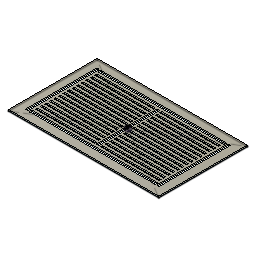
top half mount v2 (Autodesk Fusion 360 design; units mm, degrees)
Autodesk Fusion 360 part; units mm, degrees
sketch "Sketch1" plane through (0, 0, 0) normal (0, 0, 1) x (1, 0, 0)
  line L0 (115.5, -68.05) -> (-115.5, -68.05)
  line L1 (-115.5, -68.05) -> (-115.5, 68.05)
  line L2 (-115.5, 68.05) -> (115.5, 68.05)
  line L3 (115.5, 68.05) -> (115.5, -68.05)
  line L4 (115.5, -68.05) -> (-115.5, 68.05) construction
  line L5 (-115.5, -68.05) -> (115.5, 68.05) construction
  dimension "d1" = 136.1
  dimension "d2" = 231
  constraint horizontal L0
  constraint perpendicular L0 L1
  constraint parallel L0 L2
  constraint parallel L1 L3
  constraint coincident L4 origin
  constraint coincident L5 origin
  measures "d1" distance of L0.end L1.end
  measures "d2" distance of L0.start L0.end
extrude "Extrude1" add sketch "Sketch1" along normal blind 2
sketch "Sketch2" plane through (0, 0, 2) normal (0, 0, 1) x (-1, 0, 0)
  line L0 (-115.5, -68.05) -> (115.5, -68.05)
  line L1 (115.5, -68.05) -> (115.5, 68.05)
  line L2 (115.5, 68.05) -> (-115.5, 68.05)
  line L3 (-115.5, 68.05) -> (-115.5, -68.05)
  line L4 (5, -8.94) -> (95, -8.94)
  line L5 (5, -1.94) -> (95, -1.94)
  line L6 (-5, -8.94) -> (-5, -11.94)
  line L7 (2, 47) -> (-2, 47)
  line L8 (-5, -29.94) -> (-5, -32.94)
  line L9 (-5, 5.06) -> (-5, 2.06)
  line L10 (-5, -36.94) -> (-5, -39.94)
  line L11 (5, 47.06) -> (95, 47.06)
  line L12 (-5, 40.06) -> (-5, 37.06)
  line L13 (-5, 19.06) -> (-5, 16.06)
  line L14 (-95, 44.06) -> (-95, 47.06)
  arc A0 (-96, 55.06) -> (-97, 54.06) centre (-96, 54.06) ccw
  line L15 (-95, -25.94) -> (-95, -22.94)
  line L16 (-95, -39.94) -> (-95, -36.94)
  arc A1 (-100, -54.94) -> (-99, -53.94) centre (-100, -53.94) ccw
  line L17 (5, 30.06) -> (5, 33.06)
  line L18 (2, -47) -> (2, 47)
  line L19 (-95, 30.06) -> (-95, 33.06)
  line L20 (5, 44.06) -> (5, 47.06)
  arc A2 (-103, -53.94) -> (-102, -54.94) centre (-102, -53.94) ccw
  line L21 (-102, 54.94) -> (-100, 54.94)
  line L22 (5, 37.06) -> (5, 40.06)
  line L23 (-95, -46.94) -> (-95, -43.94)
  line L24 (-95.0527, 9.06) -> (-95.0527, 12.06)
  line L25 (-5, -1.94) -> (-5, -4.94)
  line L26 (5, 16.06) -> (5, 19.06)
  arc A3 (-97, -53.94) -> (-96, -54.94) centre (-96, -53.94) ccw
  line L27 (-100, -54.94) -> (-102, -54.94)
  line L28 (-95.0527, 2.06) -> (-95.0527, 5.06)
  line L29 (-97, 54.06) -> (-97, 52.06)
  line L30 (-5, -43.94) -> (-5, -46.94)
  line L31 (-97, -53.94) -> (-97, -51.94)
  line L32 (5, -4.94) -> (5, -1.94)
  line L33 (5, 23.06) -> (5, 26.06)
  line L34 (-5, -22.94) -> (-5, -25.94)
  line L35 (-2, 47) -> (-2, -47)
  line L36 (-94.8877, -18.94) -> (-94.8877, -15.94)
  line L37 (-2, 47) -> (2, -47) construction
  arc A4 (-96, -50.94) -> (-97, -51.94) centre (-96, -51.94) ccw
  line L38 (-103, -53.94) -> (-103, 53.94)
  line L39 (5, -46.94) -> (5, -43.94)
  line L40 (-95.0527, -11.94) -> (-95.0527, -8.94)
  line L41 (5, 9.06) -> (5, 12.06)
  line L42 (-95.0527, 16.06) -> (-95.0527, 19.06)
  line L43 (-95, -32.94) -> (-95, -29.94)
  line L44 (5, -39.94) -> (5, -36.94)
  line L45 (5, -18.94) -> (5, -15.94)
  arc A5 (-97, 52.06) -> (-96, 51.06) centre (-96, 52.06) ccw
  line L46 (-95, 37.06) -> (-95, 40.06)
  line L47 (-95.0527, -4.94) -> (-95.0527, -1.94)
  arc A6 (-102, 54.94) -> (-103, 53.94) centre (-102, 53.94) ccw
  line L48 (-99, 53.94) -> (-99, -53.94)
  line L49 (95, -29.94) -> (95, -32.94)
  line L50 (-94.8877, -15.94) -> (-5, -15.94)
  line L51 (-5, -25.94) -> (-95, -25.94)
  line L52 (-5, -4.94) -> (-95.0527, -4.94)
  line L53 (95, 26.06) -> (95, 23.06)
  line L54 (-5, -18.94) -> (-94.8877, -18.94)
  line L55 (-5, -11.94) -> (-95.0527, -11.94)
  line L56 (95, 33.06) -> (95, 30.06)
  arc A7 (99, -53.94) -> (100, -54.94) centre (100, -53.94) ccw
  line L57 (-5, 44.06) -> (-95, 44.06)
  line L58 (103, 53.94) -> (103, -53.94)
  line L59 (5, -25.94) -> (5, -22.94)
  arc A8 (100, 54.94) -> (99, 53.94) centre (100, 53.94) ccw
  line L60 (-95.0527, 23.06) -> (-5, 23.06)
  line L61 (97, 52.06) -> (97, 54.06)
  arc A9 (103, 53.94) -> (102, 54.94) centre (102, 53.94) ccw
  line L62 (-95.0527, 26.06) -> (-95.0527, 23.06)
  line L63 (-5, -39.94) -> (-95, -39.94)
  line L64 (5, 2.06) -> (5, 5.06)
  line L65 (-5, 47.06) -> (-5, 44.06)
  arc A10 (-99, 53.94) -> (-100, 54.94) centre (-100, 53.94) ccw
  line L66 (95, -36.94) -> (95, -39.94)
  line L67 (2, 47) -> (-2, -47) construction
  line L68 (-95.0527, 12.06) -> (-5, 12.06)
  arc A11 (97, 54.06) -> (96, 55.06) centre (96, 54.06) ccw
  line L69 (-95, -29.94) -> (-5, -29.94)
  line L70 (-95.0527, -8.94) -> (-5, -8.94)
  line L71 (95, -43.94) -> (95, -46.94)
  line L72 (-95.0527, 5.06) -> (-5, 5.06)
  line L73 (95, 19.06) -> (95, 16.06)
  line L74 (95, 12.06) -> (95, 9.06)
  line L75 (-95, -36.94) -> (-5, -36.94)
  line L76 (-5, 30.06) -> (-95, 30.06)
  line L77 (-95, -43.94) -> (-5, -43.94)
  line L78 (-5, 26.06) -> (-95.0527, 26.06)
  line L79 (-2, -47) -> (2, -47)
  line L80 (-5, 33.06) -> (-5, 30.06)
  line L81 (-5, 23.06) -> (-5, 26.06)
  line L82 (95, -46.94) -> (5, -46.94)
  line L83 (95, 44.06) -> (5, 44.06)
  line L84 (5, 12.06) -> (95, 12.06)
  line L85 (95, -39.94) -> (5, -39.94)
  line L86 (5, -15.94) -> (95, -15.94)
  line L87 (96, 55.06) -> (-96, 55.06)
  line L88 (95, -18.94) -> (5, -18.94)
  line L89 (95, 16.06) -> (5, 16.06)
  line L90 (5, 5.06) -> (95, 5.06)
  line L91 (95, 2.06) -> (5, 2.06)
  line L92 (-96, -50.94) -> (96, -50.94)
  line L93 (5, 40.06) -> (95, 40.06)
  line L94 (95, -11.94) -> (5, -11.94)
  line L95 (95, -4.94) -> (5, -4.94)
  line L96 (95, -32.94) -> (5, -32.94)
  line L97 (5, 26.06) -> (95, 26.06)
  line L98 (96, -54.94) -> (-96, -54.94)
  line L99 (95, -25.94) -> (5, -25.94)
  line L100 (95, 9.06) -> (5, 9.06)
  line L101 (95, -1.94) -> (95, -4.94)
  line L102 (5, 33.06) -> (95, 33.06)
  line L103 (95, -15.94) -> (95, -18.94)
  line L104 (5, -43.94) -> (95, -43.94)
  arc A12 (102, -54.94) -> (103, -53.94) centre (102, -53.94) ccw
  line L105 (5, -22.94) -> (95, -22.94)
  arc A13 (96, 51.06) -> (97, 52.06) centre (96, 52.06) ccw
  line L106 (-95.0527, 19.06) -> (-5, 19.06)
  line L107 (95, 23.06) -> (5, 23.06)
  line L108 (-5, 9.06) -> (-95.0527, 9.06)
  line L109 (-95, -22.94) -> (-5, -22.94)
  line L110 (95, -8.94) -> (95, -11.94)
  line L111 (-5, 16.06) -> (-95.0527, 16.06)
  line L112 (-95, 47.06) -> (-5, 47.06)
  line L113 (95, 47.06) -> (95, 44.06)
  arc A14 (97, -51.94) -> (96, -50.94) centre (96, -51.94) ccw
  line L114 (5, 19.06) -> (95, 19.06)
  line L115 (95, -22.94) -> (95, -25.94)
  line L116 (-5, 37.06) -> (-95, 37.06)
  line L117 (102, -54.94) -> (100, -54.94)
  line L118 (97, -51.94) -> (97, -53.94)
  line L119 (-95, 40.06) -> (-5, 40.06)
  line L120 (100, 54.94) -> (102, 54.94)
  line L121 (95, 40.06) -> (95, 37.06)
  line L122 (5, -36.94) -> (95, -36.94)
  line L123 (-5, -32.94) -> (-95, -32.94)
  arc A15 (96, -54.94) -> (97, -53.94) centre (96, -53.94) ccw
  line L124 (-95, 33.06) -> (-5, 33.06)
  line L125 (99, -53.94) -> (99, 53.94)
  line L126 (95, 5.06) -> (95, 2.06)
  line L127 (95, 30.06) -> (5, 30.06)
  line L128 (-5, 2.06) -> (-95.0527, 2.06)
  line L129 (-5, -46.94) -> (-95, -46.94)
  line L130 (-96, 51.06) -> (96, 51.06)
  line L131 (-95.0527, -1.94) -> (-5, -1.94)
  line L132 (5, -29.94) -> (95, -29.94)
  line L133 (5, -32.94) -> (5, -29.94)
  line L134 (5, -11.94) -> (5, -8.94)
  line L135 (-5, -15.94) -> (-5, -18.94)
  line L136 (95, 37.06) -> (5, 37.06)
  line L137 (-5, 12.06) -> (-5, 9.06)
  point P0 (103, -54.94)
  point P1 (99, -54.94)
  point P2 (-97, -50.94)
  point P3 (-97, -54.94)
  dimension "d5" = 4
  dimension "d9" = 4
  dimension "d11" = 2
  dimension "d12" = 2
  dimension "d13" = 4
  dimension "d16" = 4
  dimension "d20" = 1
  dimension "d21" = 3
  dimension "d22" = 4
  dimension "d23" = 90
  dimension "d24" = 4
  dimension "d25" = 3
  dimension "d26" = 90
  dimension "d27" = 0
  dimension "d28" = 0
  dimension "d29" = 3
  dimension "d30" = 3
  dimension "d31" = 3
  dimension "d32" = 3
  dimension "d33" = 3
  dimension "d34" = 3
  dimension "d35" = 3
  dimension "d36" = 3
  dimension "d37" = 3
  dimension "d38" = 3
  dimension "d39" = 4
  dimension "d40" = 4
  dimension "d41" = 4
  dimension "d42" = 4
  dimension "d43" = 4
  dimension "d44" = 4
  dimension "d45" = 4
  dimension "d46" = 4
  dimension "d47" = 4
  dimension "d48" = 4
  dimension "d49" = 4
  dimension "d50" = 3
  dimension "d51" = 4
  dimension "d52" = 3
  dimension "d53" = 4
  dimension "d54" = 4
  dimension "d55" = 90
  dimension "d56" = 3
  dimension "d57" = 4
  dimension "d58" = 4
  dimension "d59" = 3
  dimension "d60" = 4
  dimension "d61" = 3
  dimension "d62" = 4
  dimension "d63" = 3
  dimension "d64" = 4
  dimension "d65" = 3
  dimension "d66" = 4
  dimension "d67" = 3
  dimension "d68" = 4
  dimension "d69" = 4
  dimension "d70" = 3
  dimension "d71" = 3
  dimension "d72" = 4
  dimension "d73" = 4
  dimension "d74" = 3
  dimension "d75" = 3
  dimension "d76" = 3
  dimension "d77" = 3
  dimension "d78" = 3
  dimension "d79" = 4
  dimension "d80" = 4
  dimension "d81" = 4
  dimension "d82" = 4
  dimension "d83" = 4
  dimension "d84" = 3
  dimension "d85" = 4
  constraint horizontal L117
  constraint vertical L125
  constraint horizontal L120
  constraint vertical L58
  constraint horizontal L98
  constraint vertical L31
  constraint horizontal L92
  constraint vertical L118
  constraint horizontal L87
  constraint vertical L29
  constraint horizontal L130
  constraint vertical L61
  constraint horizontal L27
  constraint vertical L38
  constraint horizontal L21
  constraint vertical L48
  constraint tangent L98 A15
  constraint tangent L118 A15
  constraint tangent L92 A14
  constraint tangent A14 L118
  constraint equal A14 A15
  constraint coincident P0 L117
  constraint coincident P0 L58
  constraint tangent A12 L117
  constraint tangent L58 A12
  constraint equal A12 A15
  constraint coincident P1 L117
  constraint coincident P1 L125
  constraint tangent A7 L117
  constraint tangent A7 L125
  constraint equal A7 A15
  constraint tangent A9 L120
  constraint tangent L58 A9
  constraint equal A9 A15
  constraint tangent A8 L125
  constraint tangent A8 L120
  constraint equal A8 A15
  constraint tangent A13 L130
  constraint tangent L61 A13
  constraint equal A13 A15
  constraint tangent A11 L87
  constraint tangent L61 A11
  constraint equal A11 A15
  constraint tangent L29 A5
  constraint tangent A5 L130
  constraint equal A5 A15
  constraint tangent A0 L87
  constraint tangent A0 L29
  constraint equal A0 A15
  constraint tangent L21 A10
  constraint tangent L48 A10
  constraint equal A10 A15
  constraint tangent L38 A6
  constraint tangent L21 A6
  constraint equal A6 A15
  constraint tangent A2 L27
  constraint tangent A2 L38
  constraint equal A2 A15
  constraint tangent A1 L27
  constraint tangent A1 L48
  constraint equal A1 A15
  constraint coincident P3 L98
  constraint coincident P3 L31
  constraint tangent A3 L98
  constraint tangent A3 L31
  constraint equal A3 A15
  constraint coincident P2 L31
  constraint coincident P2 L92
  constraint tangent L31 A4
  constraint tangent A4 L92
  constraint equal A4 A15
  constraint horizontal L82
  constraint vertical L39
  constraint horizontal L104
  constraint vertical L71
  constraint horizontal L85
  constraint vertical L44
  constraint horizontal L122
  constraint vertical L66
  constraint horizontal L96
  constraint vertical L133
  constraint horizontal L132
  constraint vertical L49
  constraint horizontal L99
  constraint vertical L59
  constraint horizontal L105
  constraint vertical L115
  constraint horizontal L88
  constraint vertical L45
  constraint horizontal L86
  constraint vertical L103
  constraint horizontal L94
  constraint vertical L134
  constraint horizontal L4
  constraint vertical L110
  constraint horizontal L95
  constraint vertical L32
  constraint horizontal L5
  constraint vertical L101
  constraint horizontal L91
  constraint vertical L64
  constraint horizontal L90
  constraint vertical L126
  constraint horizontal L100
  constraint vertical L41
  constraint horizontal L84
  constraint vertical L74
  constraint horizontal L89
  constraint vertical L26
  constraint horizontal L114
  constraint vertical L73
  constraint horizontal L107
  constraint vertical L33
  constraint horizontal L97
  constraint vertical L53
  constraint horizontal L127
  constraint vertical L17
  constraint horizontal L102
  constraint vertical L56
  constraint horizontal L136
  constraint vertical L22
  constraint horizontal L93
  constraint vertical L121
  constraint horizontal L83
  constraint vertical L20
  constraint horizontal L11
  constraint vertical L113
  constraint horizontal L129
  constraint vertical L23
  constraint horizontal L77
  constraint vertical L30
  constraint horizontal L63
  constraint vertical L16
  constraint horizontal L75
  constraint vertical L10
  constraint horizontal L123
  constraint vertical L43
  constraint horizontal L69
  constraint vertical L8
  constraint horizontal L51
  constraint vertical L15
  constraint horizontal L109
  constraint vertical L34
  constraint horizontal L54
  constraint vertical L36
  constraint horizontal L50
  constraint vertical L135
  constraint horizontal L55
  constraint vertical L40
  constraint horizontal L70
  constraint vertical L6
  constraint horizontal L52
  constraint vertical L47
  constraint horizontal L131
  constraint vertical L25
  constraint horizontal L128
  constraint vertical L28
  constraint horizontal L72
  constraint vertical L9
  constraint horizontal L108
  constraint vertical L24
  constraint horizontal L68
  constraint vertical L137
  constraint horizontal L111
  constraint vertical L42
  constraint horizontal L106
  constraint vertical L13
  constraint horizontal L78
  constraint vertical L62
  constraint horizontal L60
  constraint vertical L81
  constraint horizontal L76
  constraint vertical L19
  constraint horizontal L124
  constraint vertical L80
  constraint horizontal L116
  constraint vertical L46
  constraint horizontal L119
  constraint vertical L12
  constraint horizontal L57
  constraint vertical L14
  constraint horizontal L112
  constraint vertical L65
  constraint horizontal L7
  constraint perpendicular L7 L35
  constraint parallel L7 L79
  constraint parallel L18 L35
  constraint coincident origin L67
  constraint coincident origin L37
  measures "d5" distance of P0 P1
  measures "d9" distance of P2 P3
  measures "d11" distance of L118 L125
  measures "d12" distance of L61 L125
  measures "d13" distance of L87 L130
  measures "d16" distance of L38 L48
  measures "d20" radius of A15
  measures "d21" distance of L71.end L71.start
  measures "d22" distance of L82 L92
  measures "d23" distance of L71.end L39.start
  measures "d24" distance of L71.start L66.end
  measures "d25" distance of L66.end L66.start
  measures "d26" distance of L66.end L44.start
  measures "d27" distance of L103 L115
  measures "d28" distance of L49 L115
  measures "d29" distance of L49.end L49.start
  measures "d30" distance of L99.start L105.end
  measures "d31" distance of L88.start L86.end
  measures "d32" distance of L4.end L94.start
  measures "d33" distance of L5.end L95.start
  measures "d34" distance of L91.start L90.end
  measures "d35" distance of L74.end L74.start
  measures "d36" distance of L73.start L73.end
  measures "d37" distance of L53.start L53.end
  measures "d38" distance of L56.end L56.start
  measures "d39" distance of L53.start L56.end
  measures "d40" distance of L73.start L53.end
  measures "d41" distance of L73.end L74.start
  measures "d42" distance of L74.end L90.end
  measures "d43" distance of L5.end L91.start
  measures "d44" distance of L95.start L4.end
  measures "d45" distance of L94.start L86.end
  measures "d46" distance of L105.end L88.start
  measures "d47" distance of L49.start L99.start
  measures "d48" distance of L66.start L49.end
  measures "d49" distance of L121.end L56.start
  measures "d50" distance of L121.end L93.end
  measures "d51" distance of L93.end L83.start
  measures "d52" distance of L83.start L11.end
  measures "d53" distance of L11 L130
  measures "d54" distance of L71.end L125
  measures "d55" distance of L30.start L23.end
  measures "d56" distance of L23.start L23.end
  measures "d57" distance of L92 L129
  measures "d58" distance of L16.start L23.end
  measures "d59" distance of L16.start L16.end
  measures "d60" distance of L43.start L16.end
  measures "d61" distance of L43.start L43.end
  measures "d62" distance of L43.end L15.start
  measures "d63" distance of L15.end L15.start
  measures "d64" distance of L54 L109
  measures "d65" distance of L36.start L36.end
  measures "d66" distance of L50 L55
  measures "d67" distance of L40.end L40.start
  measures "d68" distance of L52 L70
  measures "d69" distance of L128 L131
  measures "d70" distance of L47.start L47.end
  measures "d71" distance of L28.end L28.start
  measures "d72" distance of L72 L108
  measures "d73" distance of L42.start L24.end
  measures "d74" distance of L24.end L24.start
  measures "d75" distance of L60.start L62.start
  measures "d76" distance of L19.end L19.start
  measures "d77" distance of L46.end L46.start
  measures "d78" distance of L14.start L14.end
  measures "d79" distance of L112 L130
  measures "d80" distance of L57 L119
  measures "d81" distance of L116 L124
  measures "d82" distance of L76 L78
  measures "d83" distance of L60 L106
  measures "d84" distance of L42.start L42.end
  measures "d85" distance of L35.end L18.start
extrude "Extrude2" cut sketch "Sketch2" against normal blind 5 contours L4 L94 L110 L134 | L5 L32 L95 L101 | L6 L40 L55 L70 | L7 L18 L35 L79 | L8 L43 L69 L123 | L9 L28 L72 L128 | L10 L16 L63 L75 | L11 L20 L83 L113 | L12 L46 L116 L119 | L13 L42 L106 L111 | L14 L57 L65 L112 | A0 L29 A5 L61 A11 L87 A13 L130 | L15 L34 L51 L109 | A1 A2 L21 L27 L38 A6 L48 A10 | L17 L56 L102 L127 | L19 L76 L80 L124 | L22 L93 L121 L136 | L23 L30 L77 L129 | L24 L68 L108 L137 | L25 L47 L52 L131 | L26 L73 L89 L114 | A3 L31 A4 L92 L98 A14 L118 A15 | L33 L53 L97 L107 | L36 L50 L54 L135 | L39 L71 L82 L104 | L41 L74 L84 L100 | L44 L66 L85 L122 | L45 L86 L88 L103 | L49 L96 L132 L133 | A7 L58 A8 A9 A12 L117 L120 L125 | L59 L99 L105 L115 | L60 L62 L78 L81 | L64 L90 L91 L126
